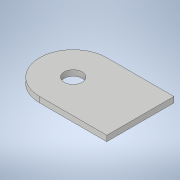
# Autodesk Inventor part: firewalltab2
Saved by Autodesk Inventor 2021 (Build 250183000, 183)
## iProperties
Created: 2020-10-29
Part Number: firewalltab2
Material: Generic
Document SubType Name: Modeling
Designer: mackeycj
Density: 1 g/cm^3
Appearance: Default
Author: mackeycj
Autodesk Inventor part; units mm, degrees
ref_plane "YZ Plane" through (0, 0, 0) normal (1, 0, 0) x (0, 1, 0)
ref_plane "XZ Plane" through (0, 0, 0) normal (0, 1, 0) x (-1, 0, 0)
ref_plane "XY Plane" through (0, 0, 0) normal (0, 0, 1) x (1, 0, 0)
sketch "Sketch1" plane through (0, 0, 0) normal (0, 1, 0) x (-1, 0, 0)
  circle A0 centre (0, 0) radius 2.5527
  circle A1 centre (0, 0) radius 9.525
  line L0 (0, 9.525) -> (-19.05, 9.525)
  line L1 (0, -9.525) -> (-19.05, -9.525)
  line L2 (-19.05, -9.525) -> (-19.05, 9.525)
  dimension "d0" = 5.1054
  dimension "d1" = 19.05
  dimension "d2" = 19.05
  dimension "d3" = 19.05
  constraints: 6 end point, 2 centre point, 2 coincident, 2 horizontal, 2 point on circle, 2 tangent
  measures "d0" diameter of A0
  measures "d1" diameter of A1
  measures "d2" distance of L0.start L0.end
  measures "d3" distance of L1.start L1.end
extrude "Extrusion1" add sketch "Sketch1" along normal mid plane 1.5875
sketch "Sketch2" plane through (0, 0, 0) normal (0, 0, 1) x (1, 0, 0)
  line L0 (0, 0) -> (31.7252, 0)
  circle A0 centre (31.7252, 0) radius 12.7
  point P0 (19.05, 0.7937)
  dimension "d7" = 25.4
  constraints: 2 end point, 1 coincident, 1 horizontal, 3 other
extrude "Extrusion2" cut sketch "Sketch2" along normal mid plane 50.8
body "Solid1"
